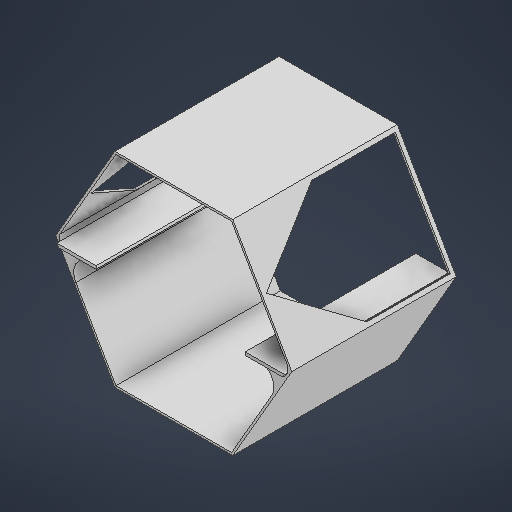
# Autodesk Inventor part: CUERPO_ABEJA
Saved by Autodesk Inventor 2026.2 (Build 302298000, 298)
## iProperties
Created: 2026-05-21
Part Number: CUERPO_ABEJA
Material: Generic
Document SubType Name: Modeling
Designer: juand
Density: 1 g/cm^3
Appearance: Default
Author: juand
Autodesk Inventor part; units mm, degrees
ref_plane "YZ Plane" through (0, 0, 0) normal (1, 0, 0) x (0, 1, 0)
ref_plane "XZ Plane" through (0, 0, 0) normal (0, 1, 0) x (-1, 0, 0)
ref_plane "XY Plane" through (0, 0, 0) normal (0, 0, 1) x (1, 0, 0)
sketch "Sketch2" plane through (0, 0, 0) normal (0, 0, 1) x (1, 0, 0)
  line L0 (28.133, -48.7278) -> (-28.133, -48.7278)
  line L1 (-28.133, -48.7278) -> (-56.266, 0)
  line L2 (-56.266, 0) -> (-28.133, 48.7278)
  line L3 (-28.133, 48.7278) -> (28.133, 48.7278)
  line L4 (28.133, 48.7278) -> (56.266, 0)
  line L5 (56.266, 0) -> (28.133, -48.7278)
  line L6 (-28.7104, 49.7278) -> (-57.4207, 0)
  line L7 (-57.4207, 0) -> (-28.7104, -49.7278)
  line L8 (-28.7104, -49.7278) -> (28.7104, -49.7278)
  line L9 (28.7104, -49.7278) -> (57.4207, 0)
  line L10 (57.4207, 0) -> (28.7104, 49.7278)
  line L11 (28.7104, 49.7278) -> (-28.7104, 49.7278)
  line L12 (0, -48.7278) -> (0, 48.7278) construction
  line L13 (-55.4, -1.5) -> (-36.266, -1.5)
  line L14 (-36.266, -1.5) -> (-36.266, -3)
  line L15 (-36.266, -3) -> (-54.534, -3)
  line L16 (55.4, -1.5) -> (36.266, -1.5)
  line L17 (36.266, -1.5) -> (36.266, -3)
  line L18 (36.266, -3) -> (54.534, -3)
  line L19 (55.4, -1.5) -> (55.4, 1.5)
  line L20 (-55.4, -1.5) -> (-55.4, 1.5)
  point P0 (0, 0)
  point P1 (0, 0)
  point P2 (54.534, -3)
  point P3 (55.4, -1.5)
  point P4 (55.4, -1.5)
  dimension "d10" = 1
  dimension "d13" = 1.5
  dimension "d14" = 20
  dimension "d15" = 1.5
  dimension "d19" = 110.8
  constraints: 42 end point, 4 point on line, 4 symmetric about line, 2 horizontal, 2 midpoint, 2 perpendicular, 1 coincident, 1 parallel, 1 vertical, 18 other
  measures "d10" distance between parallel lines of L2 L6
  measures "d13" distance between parallel lines of L15 L13
  measures "d14" horizontal distance of L1.end L13.end
  measures "d15" distance from line of L1.end L13
  measures "d19" distance of L16.start L13.start
extrude "Extrusion1" add sketch "Sketch2" along normal mid plane 80 contours L18 L17 L16 L5 | L1 L13 L14 L15 | L19 L4 L5 | L1 L2 L20 | L11 L10 L9 L8 L7 L6
extrude "Extrusion2" add sketch "Sketch2" along normal mid plane 83 contours L18 L17 L16 L5 | L1 L13 L14 L15
fillet "Fillet1" radius 8 2 edges at (-54.534, -3, 0) (54.534, -3, 0)
sketch "Sketch4" plane through (28.7104, 49.7278, 40) normal (0.8660254, 0.5, 0) x (0, 0, -1)
  line L0 (80, 0) -> (0, 0) projected
  line L1 (0, -57.4207) -> (0, 0) projected
  line L2 (80, 0) -> (80, -57.4207) projected
  line L3 (80, -57.4207) -> (0, -57.4207) projected
  line L4 (2, -2) -> (78, -2)
  line L5 (78, -2) -> (78, -55.4207)
  line L6 (78, -55.4207) -> (2, -55.4207)
  line L7 (2, -55.4207) -> (2, -2)
  line L8 (78, -28.7104) -> (40, -28.7104) construction
  line L9 (40, -28.7104) -> (40, -2) construction
  line L10 (37.4458, -2) -> (2, -28.7104)
  line L11 (37.4458, -55.4207) -> (2, -28.7104)
  point P0 (37.4458, -55.4207)
  dimension "d24" = 2
  dimension "d27" = 37
  constraints: 16 end point, 3 midpoint, 1 horizontal, 1 point on line, 1 symmetric about line, 3 other
  measures "d24" distance between parallel lines of L0 L4
  measures "d27" angle of L4 L10
extrude "Extrusion4" cut sketch "Sketch4" against normal up to surface (1 mm away) contours L4 L5 L6 L11 L10
mirror "Mirror2" about plane through (0, 0, 0) normal (1, 0, 0) of "Extrusion4"
body "Solid2"
